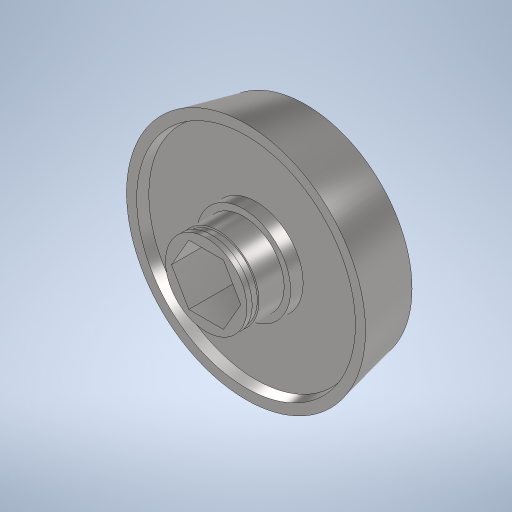
# Autodesk Inventor part: Clutch
Saved by Autodesk Inventor 2023.2 (Build 272271000, 271)
## iProperties
Created: 2024-02-03
Part Number: Clutch
Material: Stainless Steel
Document SubType Name: Modeling
Designer: Nathan Cai
Density: 8 g/cm^3
Appearance: Semi-Polished
Author: Nathan Cai
Autodesk Inventor part; units mm, degrees
ref_plane "YZ Plane" through (0, 0, 0) normal (1, 0, 0) x (0, 1, 0)
ref_plane "XZ Plane" through (0, 0, 0) normal (0, 1, 0) x (-1, 0, 0)
sketch "Sketch4" plane through (0, 0, 0) normal (0, 1, 0) x (-1, 0, 0)
  line L0 (0, 0) -> (6.5, 0) construction
  line L1 (6.5, 0) -> (6.5, -9.525)
  line L2 (6.5, -9.525) -> (0, -9.525)
  line L3 (0, -9.525) -> (0, 0)
  line L4 (0, -9.525) -> (19.05, -9.525)
  line L5 (19.05, -9.525) -> (19.05, 0) construction
  line L6 (19.05, 0) -> (0, 0)
  line L7 (0, 0) -> (0, -9.525) construction
  line L8 (19.05, 0) -> (16.9384, -9.525)
  line L9 (17.424, 0) -> (15.3123, -9.525)
  line L10 (15.6643, -7.9375) -> (6.5, -7.9375)
  line L11 (6.5, -7.9375) -> (7.5, -7.9375)
  line L12 (7.5, -7.9375) -> (7.5, -5.9375)
  line L13 (7.5, -5.9375) -> (6.5, -5.9375)
  line L14 (6.5, -5.9375) -> (6.5, -7.9375)
  line L15 (6.5, 0) -> (0, 0)
  line L16 (0, 0) -> (0, 6.35)
  line L17 (0, 6.35) -> (6.5, 6.35)
  line L18 (6.5, 6.35) -> (6.5, 0)
  line L19 (6.5, -3.175) -> (17.072, -3.175)
  line L20 (17.072, -3.175) -> (17.072, -1.5875) construction
  line L21 (17.072, -1.5875) -> (6.5, -1.5875)
  line L22 (6.5, -1.5875) -> (6.5, -3.175)
  line L23 (6.5, -3.175) -> (0, -3.175)
  line L24 (6.5, -1.5875) -> (7.5, -1.5875)
  line L25 (7.5, -1.5875) -> (7.5, 0.4125)
  line L26 (7.5, 0.4125) -> (6.5, 0.4125)
  line L27 (6.5, 0.4125) -> (6.5, -1.5875)
  line L28 (15.3123, -9.525) -> (15.3123, -3.175)
  point P0 (0, -3.175)
  point P1 (16.7201, -3.175)
  dimension "d28" = 6.5
  dimension "d30" = 19.05
  dimension "d31" = 9.525
  dimension "d32" = 12.5
  dimension "d33" = 1.5875
  dimension "d34" = 1.5875
  dimension "d36" = 1
  dimension "d37" = 2
  dimension "d53" = 6.35
  dimension "d54" = 1.5875
  dimension "d55" = 9.525
  dimension "d56" = 1
  dimension "d57" = 2
  constraints: 58 end point, 13 parallel, 11 point on line, 9 perpendicular, 6 horizontal
  measures "d28" distance of L1.end L2.end
  measures "d30" distance of L6.end L5.end
  measures "d31" distance of L5.end L4.end
  measures "d32" angle of L5 L8
  measures "d33" distance between parallel lines of L8 L9
  measures "d34" distance between parallel lines of L4 L10
  measures "d36" distance of L13.end L12.end
  measures "d37" distance of L12.end L11.end
  measures "d53" distance between parallel lines of L6 L17
  measures "d54" distance between parallel lines of L19 L21
  measures "d55" distance between parallel lines of L17 L19
  measures "d56" distance between parallel lines of L27 L25
  measures "d57" distance between parallel lines of L24 L26
revolve "Revolution1" add sketch "Sketch4" angle 360 about axis through (0, 0, -9.525) along (0, 0, 1) contours L6 L25 L21 L1 | L1 L23 L3 L6 | L18 L26 L25 L6 | L6 L16 L17 L18 | L21 L9 L19 L1 | L6 L8 L4 L9 | L19 L9 L10 L28 | L10 L9 L28
sketch "Sketch5" plane through (0, 0, 0) normal (0, 0, 1) x (1, 0, 0)
  circle A0 centre (0, 0) radius 4.7625 construction
  line L0 (0, 0) -> (0, 4.7625) construction
  line L1 (2.7496, 4.7625) -> (5.4993, 0)
  line L2 (5.4993, 0) -> (2.7496, -4.7625)
  line L3 (2.7496, -4.7625) -> (-2.7496, -4.7625)
  line L4 (-2.7496, -4.7625) -> (-5.4993, 0)
  line L5 (-5.4993, 0) -> (-2.7496, 4.7625)
  line L6 (-2.7496, 4.7625) -> (2.7496, 4.7625)
  line L7 (-2.7496, 4.7625) -> (0, 0) construction
  arc A1 (-0.9165, 4.4712) -> (-2.6268, 4.5498) centre (-1.8331, 3.175) ccw
  arc A2 (-0.9165, 4.4712) -> (0, 4.1799) centre (0, 5.7674) ccw
  arc A3 (2.6268, 4.5498) -> (0.9165, 4.4712) centre (1.8331, 3.175) ccw
  arc A4 (0, 4.1799) -> (0.9165, 4.4712) centre (0, 5.7674) ccw
  arc A5 (-4.3304, 1.4418) -> (-5.2537, 0) centre (-3.6662, 0) ccw
  arc A6 (-4.3304, 1.4418) -> (-3.6199, 2.0899) centre (-4.9947, 2.8837) ccw
  arc A7 (-3.6199, 2.0899) -> (-3.4139, 3.0293) centre (-4.9947, 2.8837) ccw
  arc A8 (-2.6268, 4.5498) -> (-3.4139, 3.0293) centre (-1.8331, 3.175) ccw
  arc A9 (-3.4139, -3.0293) -> (-2.6268, -4.5498) centre (-1.8331, -3.175) ccw
  arc A10 (-3.4139, -3.0293) -> (-3.6199, -2.0899) centre (-4.9947, -2.8837) ccw
  arc A11 (-3.6199, -2.0899) -> (-4.3304, -1.4418) centre (-4.9947, -2.8837) ccw
  arc A12 (-5.2537, 0) -> (-4.3304, -1.4418) centre (-3.6662, 0) ccw
  arc A13 (0.9165, -4.4712) -> (2.6268, -4.5498) centre (1.8331, -3.175) ccw
  arc A14 (0.9165, -4.4712) -> (0, -4.1799) centre (0, -5.7674) ccw
  arc A15 (0, -4.1799) -> (-0.9165, -4.4712) centre (0, -5.7674) ccw
  arc A16 (-2.6268, -4.5498) -> (-0.9165, -4.4712) centre (-1.8331, -3.175) ccw
  arc A17 (4.3304, -1.4418) -> (5.2537, 0) centre (3.6662, 0) ccw
  arc A18 (4.3304, -1.4418) -> (3.6199, -2.0899) centre (4.9947, -2.8837) ccw
  arc A19 (3.6199, -2.0899) -> (3.4139, -3.0293) centre (4.9947, -2.8837) ccw
  arc A20 (2.6268, -4.5498) -> (3.4139, -3.0293) centre (1.8331, -3.175) ccw
  arc A21 (3.4139, 3.0293) -> (2.6268, 4.5498) centre (1.8331, 3.175) ccw
  arc A22 (3.4139, 3.0293) -> (3.6199, 2.0899) centre (4.9947, 2.8837) ccw
  arc A23 (3.6199, 2.0899) -> (4.3304, 1.4418) centre (4.9947, 2.8837) ccw
  arc A24 (5.2537, 0) -> (4.3304, 1.4418) centre (3.6662, 0) ccw
  point P0 (-1.8331, 4.7625)
  point P1 (-3.2079, 3.9688)
  point P2 (-5.041, 0.7937)
  point P3 (-5.041, -0.7938)
  point P4 (-3.2079, -3.9687)
  point P5 (-1.8331, -4.7625)
  point P6 (1.8331, -4.7625)
  point P7 (3.2079, -3.9687)
  point P8 (5.041, -0.7937)
  point P9 (5.041, 0.7937)
  point P10 (3.2079, 3.9687)
  point P11 (1.8331, 4.7625)
  dimension "d38" = 9.525
  dimension "d47" = 1.5875
  dimension "d48" = 1.5875
  dimension "d51" = 360
  constraints: 48 point on circle, 24 centre point, 16 end point, 3 symmetric about line, 3 tangent, 2 coincident, 2 point on line, 1 line through centre, 1 midpoint, 1 vertical, 1 vertical alignment, 90 other
  measures "d47" radius of A1
  measures "d48" radius of A2
extrude "Extrusion4" cut sketch "Sketch5" along normal through all both and the other way through all
thicken "Thicken3" operation add thickness 0.0254 both sides no extend neighbours yes toward (0.9967573, -0.0804666, 0) faces at (-6.4789, 0.523, 2.3917)
ref_plane "Work Plane1" through (0, 0, 4.4125) normal (0, 0, 1) x (1, 0, 0)
sketch "Sketch6" plane through (0, 0, 4.4125) normal (0, 0, 1) x (1, 0, 0)
  circle A0 centre (0, 0) radius 6.2
  circle A1 centre (0, 0) radius 7.9375
  dimension "d43" = 12.4
  dimension "d44" = 15.875
  constraints: 2 centre point, 2 coincident
  measures "d43" diameter of A0
  measures "d44" diameter of A1
extrude "Extrusion5" cut sketch "Sketch6" along normal blind 1.1
thicken "Thicken1" operation cut thickness 0.0127 both sides no extend neighbours yes toward (0.9505525, -0.2227193, 0.2164396) faces at (-17.8624, 4.1852, -3.175)
thicken "Thicken4" operation add thickness 0.0254 both sides no extend neighbours yes toward (0, 1, 0) faces at (0.9165, 4.7625, 3.175) (-4.5827, 1.5875, 3.175) (-4.5827, -1.5875, 0) (-0.9165, -4.7625, 0) (4.5827, -1.5875, 3.175) (4.5827, 1.5875, 0)
equation "\"d34\" = d33"
equation "\"d54\" = d34"
equation "\"d55\" = d31"
equation "\"d56\" = d36"
equation "\"d57\" = d37"
equation "\"d48\" = d47"
body "Solid1"
body "Solid2"
